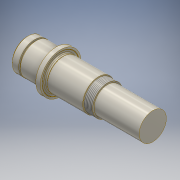
# Autodesk Inventor part: big
Saved by Autodesk Inventor 2016 (Build 200138000, 138)
## iProperties
Created: 2021-04-07
Part Number: big
Material: Типовые
Document SubType Name: Modeling
Designer: Лол
Density: 1 g/cm^3
Appearance: Титан
Author: Лол
Autodesk Inventor part; units mm, degrees
ref_plane "YZ Plane" through (0, 0, 0) normal (1, 0, 0) x (0, 1, 0)
ref_plane "XZ Plane" through (0, 0, 0) normal (0, 1, 0) x (-1, 0, 0)
ref_plane "XY Plane" through (0, 0, 0) normal (0, 0, 1) x (1, 0, 0)
sketch "Эскиз1" plane through (0, 0, 0) normal (0, 0, 1) x (1, 0, 0)
  line L0 (0, 0) -> (0, 17.5)
  line L1 (0, 17.5) -> (8.1, 17.5)
  line L2 (8.1, 17.5) -> (8.1, 15.8)
  line L3 (8.1, 15.8) -> (10, 15.8)
  line L4 (10, 15.8) -> (10, 17.5)
  line L5 (10, 17.5) -> (32, 17.5)
  line L6 (32, 17.5) -> (32, 22.5)
  line L7 (32, 22.5) -> (37, 22.5)
  line L8 (37, 22.5) -> (37, 17.5)
  line L9 (37, 17.5) -> (79, 17.5)
  line L10 (79, 17.5) -> (79, 16.5)
  line L11 (79, 16.5) -> (89, 16.5)
  line L12 (89, 16.5) -> (89, 15)
  line L13 (89, 15) -> (139, 15)
  line L14 (139, 15) -> (139, 0)
  line L15 (139, 0) -> (0, 0)
  line L16 (-27.8, 0) -> (166.8, 0) construction
  line L17 (0, -4.5) -> (0, 27) construction
  point P0 (0, 0)
  dimension "d1" = 1.9
  dimension "d2" = 10
  dimension "d3" = 22
  dimension "d4" = 5
  dimension "d5" = 42
  dimension "d6" = 10
  dimension "d7" = 50
  dimension "d12" = 0
  dimension "d13" = 1.7
  dimension "d14" = 0
  dimension "d16" = 35
  dimension "d17" = 45
  dimension "d18" = 33
  dimension "d20" = 30
  constraints: 32 end point, 12 perpendicular, 3 point on line, 1 vertical
  measures "d1" distance of L2.end L3.end
  measures "d2" distance between parallel lines of L0 L4
  measures "d3" distance of L4.end L5.end
  measures "d4" distance of L6.end L7.end
  measures "d5" distance of L8.end L9.end
  measures "d6" distance of L10.end L11.end
  measures "d7" distance of L12.end L13.end
  measures "d12" distance between parallel lines of L0 L17
  measures "d13" distance of L3.end L4.end
  measures "d14" distance between parallel lines of L15 L16
  measures "d16" diameter of L1 L16
  measures "d17" diameter of L7 L16
  measures "d18" diameter of L11 L16
  measures "d20" diameter of L13 L16
revolve "Вращение1" add sketch "Эскиз1" angle 360 about axis through (-10, 0, 0) along (1, 0, 0)
thread "Резьба1" size "M33x1.5" class "6g" standard "ANSI Metric M Profile" full length
chamfer "Фаска1" distance 1 angle 45 1 edges at (0, -17.5, 0)
sketch "Эскиз2" plane through (0, 0, 0) normal (0, 0, 1) x (1, 0, 0)
  line L0 (37, 17.5) -> (79, 17.5) construction
  line L1 (37, -22.5) -> (37, 22.5) construction
  line L2 (37, 20.55) -> (36.7, 20.25)
  line L3 (36.7, 20.25) -> (36.7, 17.25)
  line L4 (36.7, 17.25) -> (39.7, 17.25)
  line L5 (39.7, 17.25) -> (39.95, 17.5)
  line L6 (37, 20.55) -> (39.95, 20.55)
  line L7 (39.95, 20.55) -> (39.95, 17.5)
  line L8 (-27.8, 0) -> (166.8, 0) projected
  point P0 (0, 0)
  dimension "d27" = 45
  dimension "d28" = 45
  dimension "d29" = 3
  dimension "d31" = 0.3
  dimension "d32" = 0.25
  constraints: 12 end point, 4 perpendicular, 2 point on line, 1 vertical
  measures "d27" angle of L0 L5
  measures "d28" angle of L1 L2
  measures "d29" distance of L3.end L4.end
  measures "d31" distance between parallel lines of L3 L1
  measures "d32" distance between parallel lines of L0 L4
revolve "Вращение2" cut sketch "Эскиз2" angle 360 about axis through (-10, 0, 0) along (1, 0, 0)
fillet "Сопряжение1" radius 1 1 edges at (36.7, -17.25, 0)
fillet "Сопряжение2" radius 0.5 1 edges at (36.7, -20.25, 0)
fillet "Сопряжение3" radius 0.5 1 edges at (39.7, -17.25, 0)
